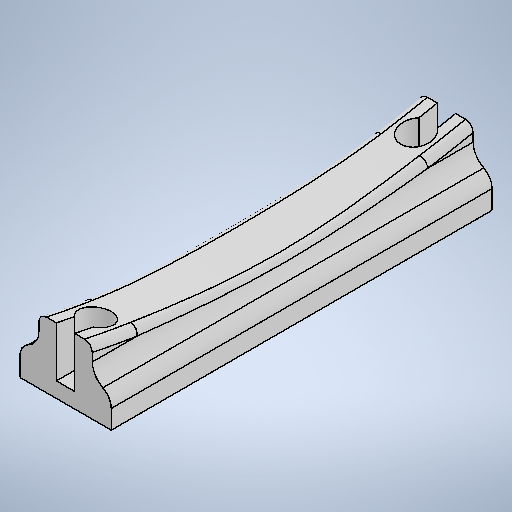
# Autodesk Inventor part: base_center
Saved by Autodesk Inventor 2026.3 (Build 303398000, 398)
## iProperties
Created: 2026-06-06
Part Number: base_center
Material: Generic
Document SubType Name: Modeling
Designer: gakut
Density: 1 g/cm^3
Appearance: Default
Author: gakut
## iProperties of the stored document base_center_3DPrint.ipt
Created: 2026-06-06
Part Number: base_center_3DPrint
Material: Generic
Document SubType Name: Modeling
Designer: gakut
Density: 1 g/cm^3
Appearance: Default
Author: gakut
Autodesk Inventor part; units mm, degrees
ref_plane "YZ Plane" through (0, 0, 0) normal (1, 0, 0) x (0, 1, 0)
ref_plane "XZ Plane" through (0, 0, 0) normal (0, 1, 0) x (-1, 0, 0)
ref_plane "XY Plane" through (0, 0, 0) normal (0, 0, 1) x (1, 0, 0)
sketch "Sketch1" plane through (0, 0, 0) normal (0, 1, 0) x (-1, 0, 0)
  line L0 (30, 125) -> (-30, 125)
  line L1 (-30, 125) -> (-30, -125)
  line L2 (-30, -125) -> (30, -125)
  line L3 (30, -125) -> (30, 125)
  line L4 (30, 125) -> (-30, -125) construction
  line L5 (-30, 125) -> (30, -125) construction
  point P0 (0, 0)
  dimension "d0" = 60
  dimension "d1" = 250
  constraints: 12 end point, 2 midpoint, 2 parallel, 1 horizontal, 1 perpendicular
  measures "d0" distance of L1.end L2.end
  measures "d1" distance of L0.end L1.end
extrude "Extrusion1" add sketch "Sketch1" along normal mid plane 20
sketch "Sketch5" plane through (0, 0, 0) normal (1, 0, 0) x (0, 1, 0)
  circle A0 centre (627.5, 0) radius 607.5
  line L0 (10, 125) -> (10, -125) projected
  line L1 (32.9992, 125) -> (10, 125)
  line L2 (32.9992, -125) -> (10, -125)
  point P0 (0, 0)
  point P1 (10, 0)
  point P2 (20, 0)
  point P3 (10, 0)
  point P4 (10, 0)
  dimension "d20" = 1215
  dimension "d21" = 10
  constraints: 4 end point, 3 midpoint, 3 point on circle, 2 horizontal alignment, 1 centre point, 1 horizontal, 1 perpendicular
  measures "d20" diameter of A0
  measures "d21" distance of point (10, 0) A0.start
extrude "Extrusion4" add sketch "Sketch5" along normal mid plane 35 contours A0 L2 L0 L1
sketch "Sketch4" plane through (0, 10, 0) normal (0, 1, 0) x (1, 0, 0)
  line L0 (-30, -125) -> (30, -125) projected
  line L1 (-6, -125) -> (6, -125)
  line L2 (6, -125) -> (6, -105)
  line L3 (6, -105) -> (-6, -105)
  line L4 (-6, -105) -> (-6, -125)
  circle A0 centre (0, -105) radius 10
  point P0 (0, 0)
  point P1 (0, -125)
  point P2 (6, -113)
  point P3 (-6, -113)
  dimension "d14" = 12
  dimension "d15" = 20
  dimension "d16" = 6
  dimension "d17" = 20
  constraints: 8 end point, 2 midpoint, 2 parallel, 1 centre point, 1 horizontal, 1 perpendicular, 1 point on line
  measures "d14" distance of L2.end L3.end
  measures "d15" distance of L3.end L1.start
  measures "d16" distance from line of point (0, -125) L4
  measures "d17" diameter of A0
extrude "Extrusion3" cut sketch "Sketch4" along normal blind 300 and the other way blind 10
sketch "Sketch6" plane through (0, 0, 0) normal (0, 1, 0) x (1, 0, 0)
  arc A0 (6, -113) -> (-6, -113) centre (0, -105) ccw projected
  point P0 (0, 0)
  constraints: 1 coincident
hole "Hole2" at (0, 0, 105) direction (0, -1, 0) diameter 3.5 end through all
mirror "Mirror1" about plane through (0, 0, 0) normal (0, 0, 1) of "Extrusion3", "Hole2"
fillet "Fillet1" radius 12.5 1 edges at (17.5, 10, 0)
fillet "Fillet2" radius 12.5 1 edges at (-17.5, 10, 0)
fillet "Fillet3" radius 5 6 edges at (17.5, 26.7308, -90.1813) (17.5, 26.7308, 90.1813) (17.7526, 20, 0) (-17.5, 26.7308, 90.1813) (-17.5, 26.7308, -90.1813) (-17.7526, 20, 0)
fillet "Fillet4" radius 10 2 edges at (30, 10, 0) (-30, 10, 0)
equation "\"d16\" = 0.5 * d14"
body "Solid1"
